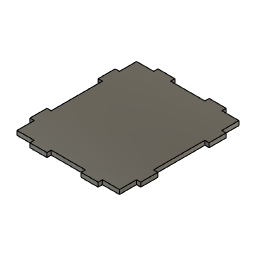
Drawer (bottem) (Autodesk Fusion 360 design; units mm, degrees)
Autodesk Fusion 360 part; units mm, degrees
sketch "Sketch1" plane through (0, 0, 0) normal (0, 0, 1) x (1, 0, 0)
  line L0 (0, 0) -> (-76.2, 0)
  line L1 (-76.2, 0) -> (-76.2, 76.2)
  line L2 (0, 76.2) -> (0, 0)
  line L3 (0, 76.2) -> (0, 88.9)
  line L4 (0, 88.9) -> (-76.2, 88.9)
  line L5 (-76.2, 88.9) -> (-76.2, 76.2)
  line L6 (-76.2, 0) -> (-63.5, 0)
  line L7 (-63.5, 0) -> (-63.5, -3.175)
  line L8 (-63.5, -3.175) -> (-50.8, -3.175)
  line L9 (-50.8, -3.175) -> (-50.8, 0)
  line L10 (-50.8, 0) -> (-38.1, 0)
  line L11 (0, 0) -> (-12.7, 0)
  line L12 (-12.7, 0) -> (-12.7, -3.175)
  line L13 (-12.7, -3.175) -> (-25.4, -3.175)
  line L14 (-25.4, -3.175) -> (-25.4, 0)
  line L15 (-76.2, 88.9) -> (-63.5, 88.9)
  line L16 (-63.5, 88.9) -> (-63.5, 92.075)
  line L17 (-63.5, 92.075) -> (-50.8, 92.075)
  line L18 (-50.8, 92.075) -> (-50.8, 88.9)
  line L19 (0, 88.9) -> (-12.7, 88.9)
  line L20 (-12.7, 88.9) -> (-12.7, 92.075)
  line L21 (-12.7, 92.075) -> (-25.4, 92.075)
  line L22 (-25.4, 92.075) -> (-25.4, 88.9)
  line L23 (-76.2, 0) -> (-76.2, 12.7)
  line L24 (-76.2, 12.7) -> (-79.375, 12.7)
  line L25 (-79.375, 12.7) -> (-79.375, 25.4)
  line L26 (-79.375, 25.4) -> (-76.2, 25.4)
  line L27 (-76.2, 88.9) -> (-76.2, 76.2)
  line L28 (-76.2, 76.2) -> (-79.375, 76.2)
  line L29 (-79.375, 76.2) -> (-79.375, 63.5)
  line L30 (-79.375, 63.5) -> (-76.2, 63.5)
  line L31 (3.175, 12.7) -> (3.175, 25.4)
  line L32 (3.175, 12.7) -> (0, 12.7)
  line L33 (3.175, 25.4) -> (0, 25.4)
  line L34 (0, 88.9) -> (0, 76.2)
  line L35 (0, 76.2) -> (3.175, 76.2)
  line L36 (3.175, 76.2) -> (3.175, 63.5)
  line L37 (3.175, 63.5) -> (0, 63.5)
  dimension "d1" = 76.2
  dimension "d2" = 76.2
  dimension "d3" = 12.7
  dimension "d4" = 3.175
  dimension "d5" = 12.7
  dimension "d6" = 12.7
  dimension "d7" = 12.7
  dimension "d8" = 3.175
  dimension "d9" = 12.7
  dimension "d10" = 12.7
  dimension "d11" = 3.175
  dimension "d12" = 12.7
  dimension "d13" = 12.7
  dimension "d14" = 3.175
  dimension "d15" = 12.7
  dimension "d16" = 12.7
  dimension "d17" = 3.175
  dimension "d18" = 12.7
  dimension "d19" = 12.7
  dimension "d20" = 3.175
  dimension "d21" = 12.7
  dimension "d24" = 12.7
  dimension "d25" = 12.7
  dimension "d26" = 3.175
  dimension "d27" = 12.7
  constraint coincident L0.start L2.end
  constraint horizontal L0
  constraint perpendicular L0 L1
  constraint perpendicular L0 L2
  constraint parallel L2 L3
  constraint perpendicular L3 L4
  constraint coincident L0 L6.end
  constraint perpendicular L6 L7
  constraint perpendicular L7 L8
  constraint coincident L0 L9.end
  constraint perpendicular L0 L9
  constraint perpendicular L9 L10
  constraint perpendicular L2 L11
  constraint perpendicular L0 L12
  constraint perpendicular L12 L13
  constraint coincident L0 L14.end
  constraint perpendicular L0 L14
  constraint perpendicular L5 L15
  constraint perpendicular L4 L16
  constraint perpendicular L16 L17
  constraint coincident L4 L18.end
  constraint perpendicular L4 L18
  constraint perpendicular L3 L19
  constraint perpendicular L4 L20
  constraint perpendicular L20 L21
  constraint coincident L4 L22.end
  constraint perpendicular L4 L22
  constraint perpendicular L0 L23
  constraint perpendicular L1 L24
  constraint perpendicular L24 L25
  constraint coincident L1 L26.end
  constraint perpendicular L1 L26
  constraint perpendicular L4 L27
  constraint perpendicular L5 L28
  constraint perpendicular L28 L29
  constraint coincident L1 L30.end
  constraint perpendicular L1 L30
  constraint coincident L2 L32.end
  constraint perpendicular L2 L32
  constraint coincident L2 L33.end
  constraint perpendicular L2 L33
  constraint perpendicular L19 L34
  constraint perpendicular L3 L35
  constraint perpendicular L35 L36
  constraint coincident L2 L37.end
  constraint perpendicular L2 L37
  measures "d1" distance of L0.start L0.end
  measures "d2" distance of L0.end L1.end
  measures "d3" distance of L2.start L3.end
  measures "d4" distance of L6.end L7.end
  measures "d5" distance of L7.end L8.end
  measures "d6" distance of L9.end L10.end
  measures "d7" distance of L0.start L11.end
  measures "d8" distance of L11.end L12.end
  measures "d9" distance of L12.end L13.end
  measures "d10" distance of L4.end L15.end
  measures "d11" distance of L15.end L16.end
  measures "d12" distance of L16.end L17.end
  measures "d13" distance of L3.end L19.end
  measures "d14" distance of L19.end L20.end
  measures "d15" distance of L20.end L21.end
  measures "d16" distance of L0.end L23.end
  measures "d17" distance of L23.end L24.end
  measures "d18" distance of L24.end L25.end
  measures "d19" distance of L4.end L1.end
  measures "d20" distance of L1.end L28.end
  measures "d21" distance of L28.end L29.end
  measures "d24" distance of L31.start L31.end
  measures "d25" distance of L3.end L2.start
  measures "d26" distance of L2.start L35.end
  measures "d27" distance of L35.end L36.end
extrude "Extrude1" add sketch "Sketch1" along normal blind 3.175
